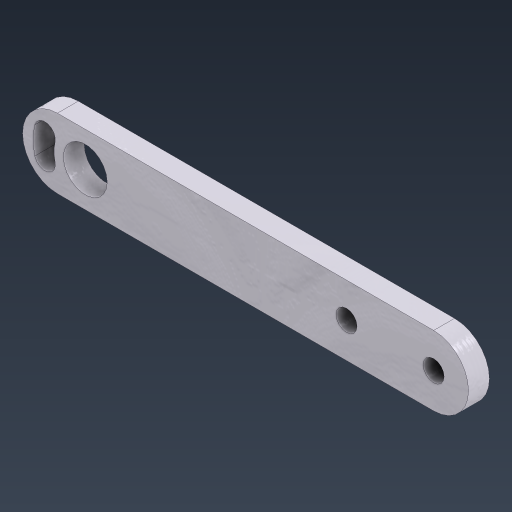
# Autodesk Inventor part: Arm2_3D
Saved by Autodesk Inventor 2023 (Build 270158000, 158)
## iProperties
Created: 2024-02-05
Part Number: Arm2_3D
Material: Aluminum 6061, Welded
Document SubType Name: Modeling
Designer: victo
Density: 2.7 g/cm^3
Appearance: Weld - Aluminum
Author: victo
Autodesk Inventor part; units mm, degrees
ref_plane "YZ Plane" through (0, 0, 0) normal (1, 0, 0) x (0, 1, 0)
ref_plane "XZ Plane" through (0, 0, 0) normal (0, 1, 0) x (-1, 0, 0)
ref_plane "XY Plane" through (0, 0, 0) normal (0, 0, 1) x (1, 0, 0)
sketch "Sketch1" plane through (0, 0, 0) normal (0, 0, 1) x (1, 0, 0)
  circle A0 centre (0, 0) radius 3.15
  line L0 (0, 0) -> (50, 0) construction
  line L1 (0, -9) -> (50, -9)
  line L2 (50, 9) -> (0, 9)
  arc A1 (0, 9) -> (0, -9) centre (0, 0) ccw
  arc A2 (50, -9) -> (50, 9) centre (50, 0) ccw
  line L3 (0, 0) -> (50, 0) construction
  circle A3 centre (50, 0) radius 1.5
  circle A4 centre (37.5, 0) radius 1.5
  circle A5 centre (-5.7956, -1.5529) radius 1.5
  circle A6 centre (-5.7956, 1.5529) radius 1.5
  line L4 (0, 0) -> (-5.7956, 1.5529) construction
  line L5 (0, 0) -> (-5.7956, -1.5529) construction
  line L6 (0, 0) -> (-9, 0) construction
  arc A7 (-4.3467, 1.1647) -> (-4.3467, -1.1647) centre (0, 0) ccw
  arc A8 (-7.2444, 1.9411) -> (-7.2444, -1.9411) centre (0, 0) ccw
  line L7 (-1.8674, 2.5368) -> (1.2741, 2.8808)
  point P0 (25, 0)
  dimension "d0" = 6.3
  dimension "d1" = 50
  dimension "d2" = 0
  dimension "d3" = 18
  dimension "d4" = 3
  dimension "d5" = 3
  dimension "d6" = 12.5
  dimension "d7" = 3
  dimension "d8" = 3
  dimension "d9" = 15
  dimension "d10" = 15
  dimension "d12" = 6
  dimension "d15" = 2.725
  dimension "d16" = -6.25
  dimension "d17" = 6
  constraints: 18 end point, 15 point on circle, 9 centre point, 6 tangent, 4 coincident, 2 horizontal, 1 collinear, 1 midpoint, 1 parallel, 1 point on line
  measures "d0" diameter of A0
  measures "d1" distance of L0.start L0.end
  measures "d2" distance between parallel lines of L0 L3
  measures "d3" diameter of A2
  measures "d4" diameter of A3
  measures "d5" diameter of A4
  measures "d6" distance of A4.centre L0.end
  measures "d7" diameter of A5
  measures "d8" diameter of A6
  measures "d9" angle of L5 L6
  measures "d10" angle of L6 L4
  measures "d12" distance of L0.start L5.end
  measures "d15" distance from line of L7 point (0, 0)
  measures "d16" angle of L0 L7
  measures "d17" distance of point (0, 0) L4.end
extrude "Extrusion1" add sketch "Sketch1" along normal blind 3
sketch "Sketch2" plane through (0, 0, 0) normal (0, 0, -1) x (-1, 0, 0)
  arc A0 (-50, 9) -> (-50, -9) centre (-50, 0) ccw projected
  line L0 (0, -9) -> (-50, -9) projected
  arc A1 (0, -9) -> (0, 9) centre (0, 0) ccw projected
  line L1 (-50, 9) -> (0, 9) projected
  circle A2 centre (-37.5, 0) radius 1.5 projected
  arc A3 (7.2444, -1.9411) -> (7.2444, 1.9411) centre (0, 0) ccw projected
  arc A4 (4.3467, -1.1647) -> (7.2444, -1.9411) centre (5.7956, -1.5529) ccw projected
  arc A5 (4.3467, -1.1647) -> (4.3467, 1.1647) centre (0, 0) ccw projected
  arc A6 (7.2444, 1.9411) -> (4.3467, 1.1647) centre (5.7956, 1.5529) ccw projected
  circle A7 centre (-50, 0) radius 1.5 projected
  circle A8 centre (0, 0) radius 3.15 projected
  line L2 (9, 5) -> (-59, 5)
  line L3 (-59, 5) -> (-59, -5)
  line L4 (-59, -5) -> (9, -5)
  line L5 (9, -5) -> (9, 5)
  circle A9 centre (-50, 0) radius 5
  point P0 (7.4833, -5)
  point P1 (-50, -5)
  point P2 (-50, 5)
  point P3 (7.4833, 5)
  dimension "d18" = 5
  dimension "d19" = 10
  dimension "d20" = 9
  dimension "d21" = 59
  constraints: 8 end point, 2 parallel, 1 centre point, 1 coincident, 1 horizontal, 1 perpendicular, 1 tangent
  measures "d18" distance from line of point (0, 0) L4
  measures "d19" distance between parallel lines of L4 L2
  measures "d20" distance from line of point (0, 0) L5
  measures "d21" distance from line of point (0, 0) L3
extrude "Extrusion2" cut sketch "Sketch2" against normal blind 5 contours L1 A1 L2 A0 | L2 A9 L4 A0 | L4 A1 L0 A0
fillet "Fillet1" radius 5 2 edges at (-7.4833, 5, 1.5) (-7.4833, -5, 1.5)
sketch "Sketch3" plane through (0, 0, 3) normal (0, 0, 1) x (1, 0, 0)
  arc A0 (-4, 5) -> (-4, -5) centre (-4, 0) ccw projected
  line L0 (-4, -5) -> (50, -5) projected
  arc A1 (50, -5) -> (50, 5) centre (50, 0) ccw projected
  line L1 (50, 5) -> (-4, 5) projected
  circle A2 centre (0, 0) radius 3.15 projected
  circle A3 centre (50, 0) radius 1.5 projected
  arc A4 (-7.2444, 1.9411) -> (-7.2444, -1.9411) centre (0, 0) ccw projected
  arc A5 (-4.3467, 1.1647) -> (-7.2444, 1.9411) centre (-5.7956, 1.5529) ccw projected
  arc A6 (-4.3467, 1.1647) -> (-4.3467, -1.1647) centre (0, 0) ccw projected
  arc A7 (-7.2444, -1.9411) -> (-4.3467, -1.1647) centre (-5.7956, -1.5529) ccw projected
  circle A8 centre (37.5, 0) radius 1.5 projected
body "Solid1"
